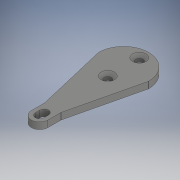
# Autodesk Inventor part: Рычаг
Saved by Autodesk Inventor 2019.3 (Build 233278000, 278)
## iProperties
Created: 2020-04-04
Part Number: Рычаг
Material: Типовые
Document SubType Name: Modeling
Designer: Admin
Density: 1 g/cm^3
Appearance: По умолчанию
Author: Admin
Autodesk Inventor part; units mm, degrees
ref_plane "YZ Plane" through (0, 0, 0) normal (1, 0, 0) x (0, 1, 0)
ref_plane "XZ Plane" through (0, 0, 0) normal (0, 1, 0) x (-1, 0, 0)
ref_plane "XY Plane" through (0, 0, 0) normal (0, 0, 1) x (1, 0, 0)
sketch "Эскиз1" plane through (0, 0, 0) normal (0, 1, 0) x (-1, 0, 0)
  arc A0 (-38, 0) -> (38, 0) centre (0, 0) ccw
  line L0 (53.2, 0) -> (-53.2, 0) projected
  line L1 (38, 0) -> (12.5, 107.5)
  line L2 (-38, 0) -> (-12.5, 107.5)
  line L3 (-12.5, 107.5) -> (-12.5, 127.5)
  line L4 (12.5, 107.5) -> (12.5, 127.5)
  arc A1 (12.5, 127.5) -> (-12.5, 127.5) centre (0, 127.5) ccw
  line L5 (0, -73.6) -> (0, 175.6) projected
  line L6 (6.5, 120.5) -> (6.5, 127.5)
  line L7 (-6.5, 120.5) -> (-6.5, 127.5)
  arc A2 (-6.5, 120.5) -> (6.5, 120.5) centre (0, 120.5) ccw
  arc A3 (6.5, 127.5) -> (-6.5, 127.5) centre (0, 127.5) ccw
  dimension "d1" = 76
  dimension "d2" = 25
  dimension "d3" = 20
  dimension "d4" = 127.5
  dimension "d5" = 7
  dimension "d6" = 13
  constraints: 12 end point, 8 point on circle, 4 centre point, 4 horizontal alignment, 3 point on line, 2 coincident, 2 equal length, 2 tangent, 2 vertical
  measures "d1" diameter of A0
  measures "d2" distance between parallel lines of L3 L4
  measures "d3" vertical distance of A1.centre L1.end
  measures "d4" distance of A1.centre point (0, 0)
  measures "d5" distance of A3.centre A2.centre
  measures "d6" distance between parallel lines of L6 L7
extrude "Выдавливание1" add sketch "Эскиз1" along normal blind 10 contours L0 L5 A0 | L2 L3 A1 L5 A3 L7 A2 L0 | L5 L0 A0 | L5 A2 L6 A3 A1 L4 L1 L0
sketch "Эскиз2" plane through (0, 10, 0) normal (0, 1, 0) x (1, 0, 0)
  point P0 (0, 0)
  point P1 (0, 24)
  point P2 (0, -24)
  dimension "d9" = 24
  dimension "d10" = 48
  constraints: 2 vertical alignment
  measures "d9" distance of point (0, 24) point (0, 0)
  measures "d10" distance of point (0, -24) point (0, 24)
hole "Отверстие1" at (0, 10, -24) at (0, 10, 24) direction (0, -1, 0) diameter 11 end through all countersink diameter 20.4 countersink angle 90 clearance for "с потайной головкой ГОСТ 12876-67" size "M10" standard "ГОСТ"
fillet "Сопряжение1" radius 2 4 edges at (12.5, 5, 107.5) (38, 5, 0) (-12.5, 5, 107.5) (-38, 5, 0)
